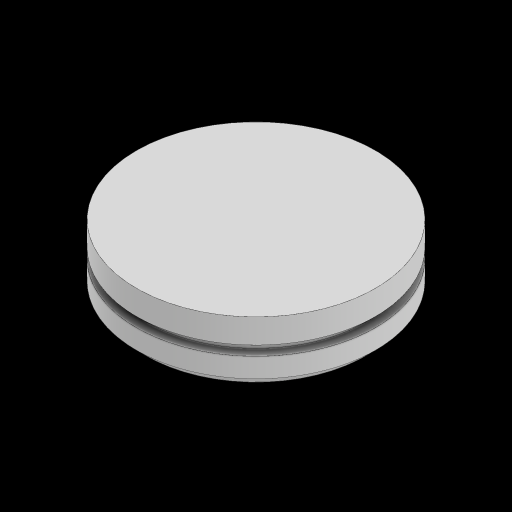
# Autodesk Inventor part: bulkhead
Saved by Autodesk Inventor 2023 (Build 270158000, 158)
## iProperties
Created: 2022-11-14
Part Number: bulkhead
Material: Generic
Document SubType Name: Modeling
Designer: user
Density: 1 g/cm^3
Appearance: Default
Author: user
Autodesk Inventor part; units mm, degrees
ref_plane "YZ Plane" through (0, 0, 0) normal (1, 0, 0) x (0, 1, 0)
ref_plane "XZ Plane" through (0, 0, 0) normal (0, 1, 0) x (-1, 0, 0)
ref_plane "XY Plane" through (0, 0, 0) normal (0, 0, 1) x (1, 0, 0)
sketch "Sketch1" plane through (0, 0, 0) normal (0, 0, 1) x (1, 0, 0)
  line L0 (0, 0) -> (-22.5, 0)
  line L1 (-24.5, 13) -> (0, 13)
  line L2 (0, 13) -> (0, 0)
  line L3 (-22.5, 0) -> (-24.5, 2)
  line L4 (-24.5, 8) -> (-22.5, 8)
  line L5 (-22.5, 8) -> (-22.5, 6)
  line L6 (-22.5, 6) -> (-24.5, 6)
  line L7 (-24.5, 6) -> (-24.5, 8)
  line L8 (-24.5, 2) -> (-24.5, 6)
  line L9 (-24.5, 8) -> (-24.5, 13)
  point P0 (-24.5, 0)
  dimension "d0" = 24.5
  dimension "d1" = 13
  dimension "d2" = 2
  dimension "d3" = 2
  dimension "d4" = 2
  dimension "d5" = 2
  dimension "d6" = 5
  dimension "d7" = 45
  constraints: 20 end point, 5 parallel, 3 perpendicular, 2 horizontal, 1 point on line
  measures "d0" distance of L1.start L1.end
  measures "d1" distance of point (-24.5, 0) L1.start
  measures "d2" distance of L0.end point (-24.5, 0)
  measures "d3" distance of L3.end point (-24.5, 0)
  measures "d4" distance of L4.start L4.end
  measures "d5" distance of L4.end L5.end
  measures "d6" distance between parallel lines of L1 L4
  measures "d7" angle of L3 L2
revolve "Revolution1" add sketch "Sketch1" angle 360 about axis through (0, 13, 0) along (0, -1, 0) contours L0 L3 L8 L6 L5 L4 L9 L1 L2
equation "\"d3\" = d2"
body "Solid1"
